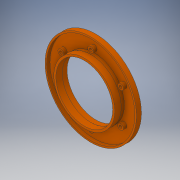
# Autodesk Inventor part: RCT-H008 Wheel Frame
Saved by Autodesk Inventor 2019 (Build 230136000, 136)
## iProperties
Created: 2019-10-01
Part Number: RCT-H008 Wheel Frame
Material: Genérico
Document SubType Name: Modeling
Designer: david
Density: 1 g/cm^3
Appearance: Valor por defecto
Author: david
Autodesk Inventor part; units mm, degrees
ref_plane "YZ Plane" through (0, 0, 0) normal (1, 0, 0) x (0, 1, 0)
ref_plane "XZ Plane" through (0, 0, 0) normal (0, 1, 0) x (-1, 0, 0)
ref_plane "XY Plane" through (0, 0, 0) normal (0, 0, 1) x (1, 0, 0)
sketch "Boceto1" plane through (0, 0, 0) normal (0, 0, 1) x (1, 0, 0)
  circle A0 centre (0, 0) radius 17.85
  circle A1 centre (0, 0) radius 28.5
  dimension "d0" = 35.7
  dimension "d89" = 57
  constraints: 2 centre point, 1 coincident
  measures "d0" diameter of A0
  measures "d89" diameter of A1
extrude "Extrusión1" add sketch "Boceto1" along normal blind 3.1
sketch "Boceto2" plane through (0, 0, 3.1) normal (0, 0, 1) x (1, 0, 0)
  circle A0 centre (0, 0) radius 19
  circle A1 centre (0, 0) radius 17.7
  dimension "d4" = 38
  dimension "d5" = 1.3
  constraints: 2 centre point, 1 coincident
  measures "d4" diameter of A0
  measures "d5" radial gap between concentric circles of A0 A1
extrude "Extrusión2" add sketch "Boceto2" along normal blind 4
sketch "Boceto3" plane through (0, 0, 0) normal (0, 0, -1) x (-1, 0, 0)
  circle A0 centre (0, 0) radius 21.5
  circle A1 centre (0, -21.5) radius 2.25
  circle A2 centre (0, -21.5) radius 0.85
  circle A3 centre (18.6195, -10.75) radius 2.25
  circle A4 centre (18.6195, -10.75) radius 0.85
  circle A5 centre (18.6195, 10.75) radius 2.25
  circle A6 centre (18.6195, 10.75) radius 0.85
  circle A7 centre (0, 21.5) radius 2.25
  circle A8 centre (0, 21.5) radius 0.85
  circle A9 centre (-18.6195, 10.75) radius 2.25
  circle A10 centre (-18.6195, 10.75) radius 0.85
  circle A11 centre (-18.6195, -10.75) radius 2.25
  circle A12 centre (-18.6195, -10.75) radius 0.85
  circle A13 centre (0, 0) radius 21.5
  circle A14 centre (0, -21.5) radius 2.25
  circle A15 centre (0, -21.5) radius 0.85
  circle A16 centre (18.6195, -10.75) radius 2.25
  circle A17 centre (18.6195, -10.75) radius 0.85
  circle A18 centre (18.6195, 10.75) radius 2.25
  circle A19 centre (18.6195, 10.75) radius 0.85
  circle A20 centre (0, 21.5) radius 2.25
  circle A21 centre (0, 21.5) radius 0.85
  circle A22 centre (-18.6195, 10.75) radius 2.25
  circle A23 centre (-18.6195, 10.75) radius 0.85
  circle A24 centre (-18.6195, -10.75) radius 2.25
  circle A25 centre (-18.6195, -10.75) radius 0.85
  dimension "d10" = 4.5
  dimension "d11" = 1.7
  dimension "d12" = 360
  dimension "d15" = 4.5
  dimension "d16" = 1.7
  dimension "d17" = 360
  constraints: 24 centre point, 12 coincident, 2 vertical alignment, 54 other
  measures "d10" diameter of A1
  measures "d11" diameter of A2
  measures "d15" diameter of A14
  measures "d16" diameter of A15
extrude "Extrusión4" cut sketch "Boceto3" against normal blind 20 contours A6 A0 | A0 A6 | A4 A0 | A0 A4 | A8 A0 | A0 A8 | A2 A0 | A0 A2 | A10 A0 | A0 A10 | A12 A0 | A0 A12
sketch "Boceto6" plane through (0, 0, 3.1) normal (0, 0, 1) x (1, 0, 0)
  circle A0 centre (0, 0) radius 21.5
  circle A1 centre (0, -21.5) radius 2.25
  circle A2 centre (0, -21.5) radius 0.85
  circle A3 centre (18.6195, -10.75) radius 2.25
  circle A4 centre (18.6195, -10.75) radius 0.85
  circle A5 centre (18.6195, 10.75) radius 2.25
  circle A6 centre (18.6195, 10.75) radius 0.85
  circle A7 centre (0, 21.5) radius 2.25
  circle A8 centre (0, 21.5) radius 0.85
  circle A9 centre (-18.6195, 10.75) radius 2.25
  circle A10 centre (-18.6195, 10.75) radius 0.85
  circle A11 centre (-18.6195, -10.75) radius 2.25
  circle A12 centre (-18.6195, -10.75) radius 0.85
  circle A13 centre (0, 0) radius 21.5
  circle A14 centre (0, -21.5) radius 2.25
  circle A15 centre (0, -21.5) radius 0.85
  circle A16 centre (18.6195, -10.75) radius 2.25
  circle A17 centre (18.6195, -10.75) radius 0.85
  circle A18 centre (18.6195, 10.75) radius 2.25
  circle A19 centre (18.6195, 10.75) radius 0.85
  circle A20 centre (0, 21.5) radius 2.25
  circle A21 centre (0, 21.5) radius 0.85
  circle A22 centre (-18.6195, 10.75) radius 2.25
  circle A23 centre (-18.6195, 10.75) radius 0.85
  circle A24 centre (-18.6195, -10.75) radius 2.25
  circle A25 centre (-18.6195, -10.75) radius 0.85
  circle A26 centre (0, 0) radius 23.75
  circle A27 centre (0, 0) radius 19 projected
  circle A28 centre (0, 0) radius 19.25
  circle A29 centre (18.6195, -10.75) radius 2.25
  dimension "d40" = 4.5
  dimension "d41" = 1.7
  dimension "d42" = 360
  dimension "d43" = 4.5
  dimension "d44" = 1.7
  dimension "d45" = 360
  constraints: 27 centre point, 14 coincident, 3 tangent, 2 vertical alignment, 54 other
  measures "d40" diameter of A1
  measures "d41" diameter of A2
  measures "d43" diameter of A14
  measures "d44" diameter of A15
shell "Vaciado1" thickness 1 removed faces 1 at (-5.8897, -22.0389, 3.1)
sketch "Boceto8" plane through (0, 0, 0) normal (0, 0, -1) x (-1, 0, 0)
  circle A0 centre (-18.6195, 10.75) radius 2.35
  circle A1 centre (-18.6195, -10.75) radius 2.35
  circle A2 centre (0, -21.5) radius 2.35
  circle A3 centre (18.6195, -10.75) radius 2.35
  circle A4 centre (18.6195, 10.75) radius 2.35
  circle A5 centre (0, 21.5) radius 2.35
  arc A6 (-18.0048, 15.6413) -> (-17.4952, 12.8136) centre (-16.6131, 14.4323) ccw
  arc A7 (-17.4952, 12.8136) -> (-13.6965, 13.3839) centre (-15.9726, 15.6079) ccw
  arc A8 (-19.8444, -8.7445) -> (-18.439, -5.1696) centre (-21.5031, -6.0287) ccw
  arc A9 (-22.5482, -7.772) -> (-19.8444, -8.7445) centre (-20.8053, -7.1712) ccw
  arc A10 (-2.3493, -21.558) -> (-4.7425, -18.5535) centre (-5.5306, -21.6366) ccw
  arc A11 (-4.5434, -23.4133) -> (-2.3493, -21.558) centre (-4.1922, -21.6035) ccw
  arc A12 (17.4952, -12.8136) -> (13.6965, -13.3839) centre (15.9726, -15.6079) ccw
  arc A13 (18.0048, -15.6413) -> (17.4952, -12.8136) centre (16.6131, -14.4323) ccw
  arc A14 (19.8444, 8.7445) -> (18.439, 5.1696) centre (21.5031, 6.0287) ccw
  arc A15 (22.5482, 7.772) -> (19.8444, 8.7445) centre (20.8053, 7.1712) ccw
  arc A16 (2.3493, 21.558) -> (4.7425, 18.5535) centre (5.5306, 21.6366) ccw
  arc A17 (4.5434, 23.4133) -> (2.3493, 21.558) centre (4.1922, 21.6035) ccw
  line L0 (0, 0) -> (-2.3493, 0) construction
  arc A18 (-18.439, 5.1696) -> (-19.8444, 8.7445) centre (-21.5031, 6.0287) ccw
  arc A19 (-19.8444, 8.7445) -> (-22.5482, 7.772) centre (-20.8053, 7.1712) ccw
  arc A20 (-13.6965, -13.3839) -> (-17.4952, -12.8136) centre (-15.9726, -15.6079) ccw
  arc A21 (-17.4952, -12.8136) -> (-18.0048, -15.6413) centre (-16.6131, -14.4323) ccw
  arc A22 (4.7425, -18.5535) -> (2.3493, -21.558) centre (5.5306, -21.6366) ccw
  arc A23 (2.3493, -21.558) -> (4.5434, -23.4133) centre (4.1922, -21.6035) ccw
  arc A24 (18.439, -5.1696) -> (19.8444, -8.7445) centre (21.5031, -6.0287) ccw
  arc A25 (19.8444, -8.7445) -> (22.5482, -7.772) centre (20.8053, -7.1712) ccw
  arc A26 (13.6965, 13.3839) -> (17.4952, 12.8136) centre (15.9726, 15.6079) ccw
  arc A27 (17.4952, 12.8136) -> (18.0048, 15.6413) centre (16.6131, 14.4323) ccw
  arc A28 (-4.7425, 18.5535) -> (-2.3493, 21.558) centre (-5.5306, 21.6366) ccw
  arc A29 (-2.3493, 21.558) -> (-4.5434, 23.4133) centre (-4.1922, 21.6035) ccw
  arc A30 (-4.7425, 18.5535) -> (-13.6965, 13.3839) centre (0, 0) ccw
  arc A31 (-4.5434, 23.4133) -> (-18.0048, 15.6413) centre (0, 0) ccw
  arc A32 (-18.439, 5.1696) -> (-18.439, -5.1696) centre (0, 0) ccw
  arc A33 (-22.5482, 7.772) -> (-22.5482, -7.772) centre (0, 0) ccw
  arc A34 (-13.6965, -13.3839) -> (-4.7425, -18.5535) centre (0, 0) ccw
  arc A35 (-18.0048, -15.6413) -> (-4.5434, -23.4133) centre (0, 0) ccw
  arc A36 (4.5434, -23.4133) -> (18.0048, -15.6413) centre (0, 0) ccw
  arc A37 (4.7425, -18.5535) -> (13.6965, -13.3839) centre (0, 0) ccw
  arc A38 (19.15, 0) -> (18.439, 5.1696) centre (0, 0) ccw
  arc A39 (13.6965, 13.3839) -> (4.7425, 18.5535) centre (0, 0) ccw
  arc A40 (22.5482, -7.772) -> (22.5482, 7.772) centre (0, 0) ccw
  arc A41 (18.0048, 15.6413) -> (4.5434, 23.4133) centre (0, 0) ccw
  arc A42 (-4.7425, 18.5535) -> (-13.6965, 13.3839) centre (0, 0) ccw
  arc A43 (-18.439, 5.1696) -> (-18.439, -5.1696) centre (0, 0) ccw
  arc A44 (13.6965, 13.3839) -> (4.7425, 18.5535) centre (0, 0) ccw
  arc A45 (18.439, -5.1696) -> (18.439, 5.1696) centre (0, 0) ccw
  arc A46 (-13.6965, -13.3839) -> (-4.7425, -18.5535) centre (0, 0) ccw
  arc A47 (4.7425, -18.5535) -> (13.6965, -13.3839) centre (0, 0) ccw
  line L1 (0, 17.85) -> (0, 18.5535) construction
  line L2 (0, 18.5535) -> (1, 18.5535) construction
  line L3 (1, 18.5535) -> (-1, 18.5535)
  line L4 (-1, 18.5535) -> (-2.8826, 19.8717)
  line L5 (-1, 18.5535) -> (1.2982, 18.5535) construction
  line L6 (1, 18.5535) -> (2.8826, 19.8717)
  line L7 (-16.5678, 8.4107) -> (-18.6507, 7.4394)
  line L8 (-15.5678, 10.1428) -> (-16.5678, 8.4107)
  line L9 (-15.5678, 10.1428) -> (-15.7681, 12.4322)
  line L10 (-15.5678, -10.1428) -> (-15.7681, -12.4322)
  line L11 (-16.5678, -8.4107) -> (-15.5678, -10.1428)
  line L12 (-16.5678, -8.4107) -> (-18.6507, -7.4394)
  line L13 (1, -18.5535) -> (2.8826, -19.8717)
  line L14 (-1, -18.5535) -> (1, -18.5535)
  line L15 (-1, -18.5535) -> (-2.8826, -19.8717)
  line L16 (16.5678, -8.4107) -> (18.6507, -7.4394)
  line L17 (15.5678, -10.1428) -> (16.5678, -8.4107)
  line L18 (15.5678, -10.1428) -> (15.7681, -12.4322)
  line L19 (15.5678, 10.1428) -> (15.7681, 12.4322)
  line L20 (16.5678, 8.4107) -> (15.5678, 10.1428)
  line L21 (16.5678, 8.4107) -> (18.6507, 7.4394)
  circle A48 centre (0, 21.5) radius 0.85
  circle A49 centre (0, 21.5) radius 0.85 projected
  circle A50 centre (-18.6195, 10.75) radius 0.85
  circle A51 centre (-18.6195, -10.75) radius 0.85
  circle A52 centre (0, -21.5) radius 0.85
  circle A53 centre (18.6195, -10.75) radius 0.85
  circle A54 centre (18.6195, 10.75) radius 0.85
  circle A55 centre (0, 0) radius 17.85
  circle A56 centre (0, 0) radius 17.85 projected
  dimension "d61" = 4.7
  dimension "d64" = 360
  dimension "d68" = 360
  dimension "d72" = 360
  dimension "d74" = 1
  dimension "d75" = 2
  dimension "d76" = 145
  dimension "d79" = 360
  dimension "d83" = 360
  constraints: 85 point on circle, 54 centre point, 44 end point, 6 coincident, 6 symmetric about line, 2 horizontal, 2 point on line, 1 concentric, 1 equal length, 1 perpendicular, 1 vertical, 1 vertical alignment, 163 other
  measures "d74" distance of L1.end L2.end
  measures "d75" distance of L2.end L3.end
  measures "d76" angle of L5 L4
extrude "Extrusión7" cut sketch "Boceto8" against normal blind 0.5 contours A6 A31 A29 A28 A30 A7 | A18 A32 A8 A9 A33 A19 | A17 A41 A27 A26 A39 A16 A5 | A20 A34 A10 A11 A35 A21 | A15 A40 A25 A24 A45 A38 A14 | A22 A37 A12 A13 A36 A23 A2
extrude "Extrusión8" cut sketch "Boceto8" against normal blind 0.7 contours A0 | A5 | A1 | A4 | A2 | A3
